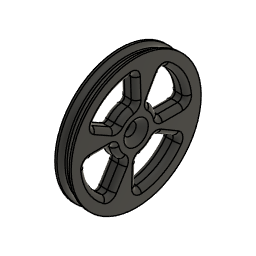
c9890e87-f5de-4b3a-b40a-a6f27797a13e (Autodesk Fusion 360 design; units mm, degrees)
Autodesk Fusion 360 part; units mm, degrees
sketch "Esboço3" plane through (0, 0, 0) normal (1, 0, 0) x (0, 1, 0)
  circle A0 centre (82.9895, -0.0021) radius 16
  circle A1 centre (82.9895, -0.0021) radius 3.6
  circle A2 centre (82.9895, -0.0021) radius 1.5
  line L0 (86.3633, 5.4063) -> (88.8299, 9.8225)
  line L1 (89.3869, 0.1483) -> (94.4318, 0.1483)
  line L2 (82.9776, 6.4513) -> (82.8139, 11.4703)
  line L3 (77.5685, 3.3629) -> (73.1649, 5.8448)
  line L4 (76.5936, -0.1572) -> (71.548, -0.1539)
  line L5 (79.7382, -5.5625) -> (77.1211, -9.8536)
  line L6 (83.249, -6.3492) -> (83.0977, -11.4188)
  line L7 (88.4805, -3.3159) -> (92.8177, -5.8791)
  arc A3 (88.4027, 0.9713) -> (86.583, 4.1617) centre (82.9895, -0.0021) ccw
  arc A4 (95.4268, 1.2483) -> (90.2867, 10.1468) centre (82.9895, -0.0021) ccw
  arc A5 (84.1936, -12.444) -> (93.1193, -7.3259) centre (82.9895, -0.0021) ccw
  arc A6 (84.0549, -5.398) -> (87.2052, -3.5345) centre (82.9895, -0.0021) ccw
  arc A7 (81.7122, 12.4324) -> (72.8443, 7.3002) centre (82.9895, -0.0021) ccw
  arc A8 (70.5524, -1.254) -> (75.6828, -10.1442) centre (82.9895, -0.0021) ccw
  arc A9 (82.1338, 5.4309) -> (78.818, 3.5823) centre (82.9895, -0.0021) ccw
  arc A10 (77.5771, -0.9795) -> (79.516, -4.2665) centre (82.9895, -0.0021) ccw
  arc A11 (82.8139, 11.4703) -> (81.7122, 12.4324) centre (81.8144, 11.4377) ccw
  arc A12 (82.1338, 5.4309) -> (82.9776, 6.4513) centre (81.9782, 6.4187) ccw
  arc A13 (77.5685, 3.3629) -> (78.818, 3.5823) centre (78.0595, 4.234) ccw
  arc A14 (72.8443, 7.3002) -> (73.1649, 5.8448) centre (73.6559, 6.716) ccw
  arc A15 (71.548, -0.1539) -> (70.5524, -1.254) centre (71.5473, -1.1539) ccw
  arc A16 (77.5771, -0.9795) -> (76.5936, -0.1572) centre (76.593, -1.1572) ccw
  arc A17 (79.7382, -5.5625) -> (79.516, -4.2665) centre (78.8845, -5.0418) ccw
  arc A18 (75.6828, -10.1442) -> (77.1211, -9.8536) centre (76.2674, -9.3329) ccw
  arc A19 (84.0549, -5.398) -> (83.249, -6.3492) centre (84.2485, -6.379) ccw
  arc A20 (88.4805, -3.3159) -> (87.2052, -3.5345) centre (87.9717, -4.1768) ccw
  arc A21 (93.1193, -7.3259) -> (92.8177, -5.8791) centre (92.3089, -6.74) ccw
  arc A22 (83.0977, -11.4188) -> (84.1936, -12.444) centre (84.0973, -11.4487) ccw
  arc A23 (94.4318, 0.1483) -> (95.4268, 1.2483) centre (94.4318, 1.1483) ccw
  arc A24 (90.2867, 10.1468) -> (88.8299, 9.8225) centre (89.7029, 9.3349) ccw
  arc A25 (86.3633, 5.4063) -> (86.583, 4.1617) centre (87.2363, 4.9187) ccw
  arc A26 (88.4027, 0.9713) -> (89.3869, 0.1483) centre (89.3869, 1.1483) ccw
  line L8 (85.8395, 2.8479) -> (80.1395, 2.8479)
  line L9 (80.1395, 2.8479) -> (80.1395, -2.8521)
  line L10 (80.1395, -2.8521) -> (85.8395, -2.8521)
  line L11 (85.8395, -2.8521) -> (85.8395, 2.8479)
  line L12 (85.8395, 2.8479) -> (80.1395, -2.8521) construction
  line L13 (80.1395, 2.8479) -> (85.8395, -2.8521) construction
  circle A27 centre (82.9895, -0.0021) radius 15.25
  point P0 (82.9895, -0.0021)
  dimension "d388_2" = 32
  dimension "d389_2" = 7.2
  dimension "d390_2" = 3
  dimension "d391_2" = 11
  dimension "d392_2" = 25
  dimension "d393_2" = 1
  dimension "d394_1" = 5.7
  dimension "d395_1" = 5.7
  dimension "d431" = 30.5
  constraint concentric A0 A7
  constraint concentric A7 A9
  constraint concentric A1 A9
  constraint concentric A1 A2
  constraint horizontal L1
  constraint concentric A3 A9
  constraint concentric A4 A7
  constraint concentric A5 A7
  constraint concentric A6 A9
  constraint concentric A7 A8
  constraint concentric A9 A10
  constraint tangent A7 A11
  constraint tangent L2 A11
  constraint tangent L2 A12
  constraint tangent A9 A12
  constraint equal A11 A12
  constraint tangent A9 A13
  constraint tangent L3 A13
  constraint equal A11 A13
  constraint tangent L3 A14
  constraint tangent A7 A14
  constraint equal A11 A14
  constraint tangent L4 A15
  constraint tangent A8 A15
  constraint equal A11 A15
  constraint tangent L4 A16
  constraint tangent A10 A16
  constraint equal A11 A16
  constraint tangent A10 A17
  constraint tangent L5 A17
  constraint equal A11 A17
  constraint tangent L5 A18
  constraint tangent A8 A18
  constraint equal A11 A18
  constraint tangent L6 A19
  constraint tangent A6 A19
  constraint equal A11 A19
  constraint tangent A6 A20
  constraint tangent L7 A20
  constraint equal A11 A20
  constraint tangent L7 A21
  constraint tangent A5 A21
  constraint equal A11 A21
  constraint tangent A5 A22
  constraint tangent L6 A22
  constraint equal A11 A22
  constraint tangent L1 A23
  constraint tangent A4 A23
  constraint equal A11 A23
  constraint tangent A4 A24
  constraint tangent L0 A24
  constraint equal A11 A24
  constraint tangent L0 A25
  constraint tangent A3 A25
  constraint equal A11 A25
  constraint tangent A3 A26
  constraint tangent L1 A26
  constraint equal A11 A26
  constraint horizontal L8
  constraint perpendicular L8 L9
  constraint parallel L8 L10
  constraint parallel L9 L11
  constraint coincident L12 P0
  constraint coincident L13 P0
  constraint coincident P0 A0.centre
  constraint equal A4 A7
  constraint equal A5 A7
  constraint equal A7 A8
  constraint concentric A9 A27
  constraint equal A3 A9
  constraint equal A6 A9
  constraint equal A9 A10
  measures "d388_2" diameter of A0
  measures "d389_2" diameter of A1
  measures "d390_2" diameter of A2
  measures "d391_2" diameter of A9
  measures "d392_2" diameter of A7
  measures "d393_2" radius of A11
  measures "d394_1" distance of L9.end L10.end
  measures "d395_1" distance of L8.end L9.end
  measures "d431" diameter of A27
extrude "Extrusão1" add sketch "Esboço3" along normal blind 4 contours A0 | A1 L11 | A1 L8 L9 L10 L11 | A1 L8 L11 | A1 L10 L11 | A1 L8 | A1 L10 | A1 L8 L9 | A1 L9 L10 | A1 L9 | A27
extrude "Extrusão2" cut sketch "Esboço3" along normal blind 1 contours A1 L8 L9 L10 L11
fillet "Arredondamento1" radius 1.2 64 edges at (4, 75.3667, 4.6039) (4, 72.6793, 6.5009) (4, 76.7283, 10.8167) (4, 82.4722, 12.1908) (4, 82.8958, 8.9608) (4, 82.7488, 5.7814) (4, 80.3113, 4.8017) (4, 78.2325, 3.2491) (4, 87.5966, 7.6144) (4, 89.4856, 10.311) (4, 93.8135, 6.2502) (4, 95.1735, 0.4775) (4, 91.9094, 0.1483) (4, 88.7454, 0.3812) (4, 87.767, 2.7229) (4, 86.2515, 4.7449) (4, 78.4297, -7.708) (4, 76.4655, -10.3131) (4, 72.163, -6.25) (4, 70.8059, -0.4829) (4, 74.0708, -0.1556) (4, 77.2344, -0.3901) (4, 78.2523, -2.7966) (4, 79.8701, -4.8728) (4, 90.6491, -4.5975) (4, 93.2879, -6.5359) (4, 89.2074, -10.8459) (4, 83.4141, -12.1789) (4, 83.1733, -8.884) (4, 83.4855, -5.7326) (4, 85.7896, -4.736) (4, 87.8028, -3.1912) (0, 90.6491, -4.5975) (0, 93.2879, -6.5359) (0, 89.2074, -10.8459) (0, 83.4141, -12.1789) (0, 83.1733, -8.884) (0, 83.4855, -5.7326) (0, 85.7896, -4.736) (0, 87.8028, -3.1912) (0, 72.163, -6.25) (0, 70.8059, -0.4829) (0, 74.0708, -0.1556) (0, 77.2344, -0.3901) (0, 78.2523, -2.7966) (0, 79.8701, -4.8728) (0, 78.4297, -7.708) (0, 76.4655, -10.3131) (0, 87.5966, 7.6144) (0, 89.4856, 10.311) (0, 93.8135, 6.2502) (0, 95.1735, 0.4775) (0, 91.9094, 0.1483) (0, 88.7454, 0.3812) (0, 87.767, 2.7229) (0, 86.2515, 4.7449) (0, 80.3113, 4.8017) (0, 78.2325, 3.2491) (0, 75.3667, 4.6039) (0, 72.6793, 6.5009) (0, 76.7283, 10.8167) (0, 82.4722, 12.1908) (0, 82.8958, 8.9608) (0, 82.7488, 5.7814)
chamfer "Chanfro1" distance 1.5 angle 45 1 edges at (4, 81.591, 0.5403)
extrude "Extrusão3" cut sketch "Esboço3" along normal blind 0.5 and the other way blind -3.5 contours A0
fillet "Arredondamento2" radius 1.4 2 edges at (3.5, 68.7715, 5.5125) (0.5, 68.7715, 5.5125)
